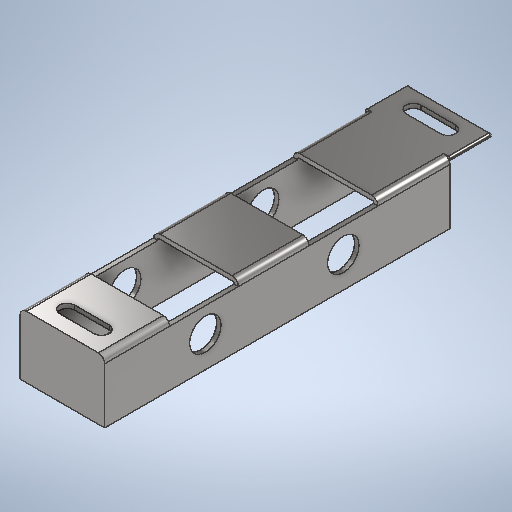
# Autodesk Inventor part: CASQUILLO RUEDA DE CORREDERA
Saved by Autodesk Inventor 2025 (Build 290162000, 162)
## iProperties
Created: 2026-02-25
Part Number: CASQUILLO RUEDA DE CORREDERA
Material: Acero inoxidable
Document SubType Name: Modeling
Designer: Frank
Density: 8 g/cm^3
Appearance: Semipulido
Author: Frank
Autodesk Inventor part; units mm, degrees
ref_plane "YZ Plane" through (0, 0, 0) normal (1, 0, 0) x (0, 1, 0)
ref_plane "XZ Plane" through (0, 0, 0) normal (0, 1, 0) x (-1, 0, 0)
ref_plane "XY Plane" through (0, 0, 0) normal (0, 0, 1) x (1, 0, 0)
sketch "Boceto1" plane through (0, 0, 0) normal (0, 0, 1) x (1, 0, 0)
  line L0 (0, 0) -> (0, 19.6)
  line L1 (0, 19.6) -> (-26.8, 19.6)
  line L2 (-26.8, 19.6) -> (-26.8, 0)
  line L3 (-25.4, 0) -> (-25.4, 18.2)
  line L4 (-25.4, 18.2) -> (-1.4, 18.2)
  line L5 (-1.4, 18.2) -> (-1.4, 0)
  line L6 (-26.8, 0) -> (-25.4, 0)
  line L7 (-1.4, 0) -> (0, 0)
  dimension "d1" = 19.6
  dimension "d2" = 1.4
  dimension "d4" = 26.8
  constraints: 16 end point, 4 perpendicular, 1 coincident, 1 collinear, 1 horizontal, 1 vertical, 2 other
  measures "d1" distance of L1.end L2.end
  measures "d2" distance between parallel lines of L4 L1
  measures "d4" distance of L0.end L1.end
extrude "Extrusión1" add sketch "Boceto1" against normal blind 108.4
fillet "Empalme1" radius 2 2 edges at (0, 19.6, -54.2) (-26.8, 19.6, -54.2)
ref_plane "Plano de trabajo1" through (0, 0, -108.4) normal (0, 0, -1) x (-1, 0, 0)
sketch "Boceto2" plane through (0, 0, -108.4) normal (0, 0, -1) x (-1, 0, 0)
  line L0 (0, 19.6) -> (26.8, 19.6)
  line L1 (26.8, 19.6) -> (26.8, 18.2)
  line L2 (26.8, 18.2) -> (0, 18.2)
  line L3 (0, 18.2) -> (0, 19.6)
  line L4 (26.8, 0) -> (26.8, 17.6) projected
  line L5 (0, 17.6) -> (0, 0) projected
  point P0 (1.4, 18.2)
  point P1 (2, 19.6)
  constraints: 8 end point, 2 collinear, 2 parallel, 2 point on line, 1 horizontal, 1 perpendicular
extrude "Extrusión2" add sketch "Boceto2" along normal blind 13.3
fillet "Empalme2" radius 0.5 1 edges at (-26.8, 18.2, -115.05)
fillet "Empalme3" radius 0.5 3 edges at (-26.8, 19.6, -115.05) (0, 19.6, -115.05) (0, 18.2, -115.05)
fillet "Empalme4" radius 0.5 8 edges at (-26.8, 18.9, -121.7) (-26.6536, 18.3464, -121.7) (-13.4, 18.2, -121.7) (-0.1464, 18.3464, -121.7) (0, 18.9, -121.7) (-0.1464, 19.4536, -121.7) (-13.4, 19.6, -121.7) (-26.6536, 19.4536, -121.7)
sketch "Boceto3" plane through (-24.8, 19.6, 0) normal (0, 1, 0) x (1, 0, 0)
  line L0 (5.91, 115.72) -> (16.89, 115.72) construction
  line L1 (5.91, 113.34) -> (16.89, 113.34)
  line L2 (16.89, 118.1) -> (5.91, 118.1)
  arc A0 (5.91, 118.1) -> (5.91, 113.34) centre (5.91, 115.72) ccw
  arc A1 (16.89, 113.34) -> (16.89, 118.1) centre (16.89, 115.72) ccw
  line L3 (-2, 121.2) -> (-2, 108.4) projected
  line L4 (24.3, 121.7) -> (-1.5, 121.7) projected
  line L5 (16.89, 5.98) -> (5.91, 5.98) construction
  line L6 (16.89, 3.6) -> (5.91, 3.6)
  line L7 (5.91, 8.36) -> (16.89, 8.36)
  arc A2 (16.89, 3.6) -> (16.89, 8.36) centre (16.89, 5.98) ccw
  arc A3 (5.91, 8.36) -> (5.91, 3.6) centre (5.91, 5.98) ccw
  line L8 (22.8, 0) -> (0, 0) projected
  line L9 (24.8, 0) -> (24.8, 108.4) projected
  point P0 (11.4, 115.72)
  point P1 (19.27, 115.72)
  point P2 (3.53, 115.72)
  point P3 (11.4, 5.98)
  point P4 (19.27, 5.98)
  point P5 (3.53, 5.98)
  dimension "d14" = 15.74
  dimension "d15" = 4.76
  dimension "d16" = 5.53
  dimension "d19" = 3.6
  dimension "d20" = 3.6
  dimension "d21" = 4.76
  dimension "d22" = 15.74
  dimension "d23" = 5.53
  constraints: 16 end point, 12 point on circle, 8 tangent, 4 centre point, 2 horizontal, 2 midpoint, 2 parallel
  measures "d14" distance of point (19.27, 115.72) point (3.53, 115.72)
  measures "d15" distance between parallel lines of L2 L1
  measures "d16" distance from line of L3 point (3.53, 115.72)
  measures "d19" distance between parallel lines of L4 L2
  measures "d20" distance between parallel lines of L8 L6
  measures "d21" distance between parallel lines of L6 L7
  measures "d22" distance of point (19.27, 5.98) point (3.53, 5.98)
  measures "d23" distance from line of L9 point (19.27, 5.98)
extrude "Extrusión3" cut sketch "Boceto3" against normal through all
ref_plane "Plano de trabajo2" through (0, 0, 0) normal (0, 0, 1) x (1, 0, 0)
sketch "Boceto4" plane through (0, 0, 0) normal (0, 0, 1) x (1, 0, 0)
  line L0 (0, 0) -> (0, 17.6) projected
  line L1 (-26.8, 19.6) -> (0, 19.6)
  line L2 (0, 19.6) -> (0, 0)
  line L3 (0, 0) -> (-26.8, 0)
  line L4 (-26.8, 0) -> (-26.8, 19.6)
  constraints: 8 end point, 2 parallel, 1 horizontal, 1 perpendicular
extrude "Extrusión4" add sketch "Boceto4" along normal blind 1
fillet "Empalme5" radius 2 2 edges at (0, 19.6, 0.5) (-26.8, 19.6, 0.5)
sketch "Boceto5" plane through (0, 0, -108.4) normal (1, 0, 0) x (0, 0, -1)
  circle A0 centre (-77.5, 9.8) radius 5
  circle A1 centre (-33.8, 9.8) radius 5
  line L0 (-109.4, 0) -> (-109.4, 17.6) projected
  line L1 (0, 0) -> (-109.4, 0) projected
  point P0 (-108.4, 0)
  dimension "d28" = 43.7
  dimension "d29" = 10
  dimension "d30" = 10
  dimension "d31" = 31.9
  dimension "d32" = 9.8
  dimension "d33" = 9.8
  constraints: 2 centre point
  measures "d28" distance of A1.centre A0.centre
  measures "d29" diameter of A0
  measures "d30" diameter of A1
  measures "d31" distance from line of L0 A0.centre
  measures "d32" distance from line of L1 A0.centre
  measures "d33" distance from line of L1 A1.centre
extrude "Extrusión5" cut sketch "Boceto5" against normal through all
ref_plane "Plano de trabajo3" through (-26.3, 19.6, -121.2) normal (0, 1, 0) x (1, 0, 0)
sketch "Boceto7" plane through (-26.3, 19.6, -121.2) normal (0, 1, 0) x (1, 0, 0)
  line L0 (26.3, -35.6145) -> (-0.5, -35.6145)
  line L1 (-0.5, -35.6145) -> (-0.5, -57.4145)
  line L2 (-0.5, -57.4145) -> (26.3, -57.4145)
  line L3 (26.3, -57.4145) -> (26.3, -35.6145)
  line L4 (26.3, -79.8455) -> (-0.5, -79.8455)
  line L5 (-0.5, -79.8455) -> (-0.5, -101.6455)
  line L6 (-0.5, -101.6455) -> (26.3, -101.6455)
  line L7 (26.3, -101.6455) -> (26.3, -79.8455)
  line L8 (26.3, -122.2) -> (26.3, -12.8) projected
  line L9 (-0.5, -12.8) -> (-0.5, -122.2) projected
  point P0 (26.3, -121.2)
  dimension "d37" = 21.8
  dimension "d38" = 21.8
  constraints: 16 end point, 4 parallel, 4 point on line, 2 horizontal, 2 perpendicular
  measures "d37" distance of L4.end L5.end
  measures "d38" distance of L0.end L1.end
extrude "Extrusión6" cut sketch "Boceto7" against normal blind 2 contours L3 L2 L1 L0 | L7 L6 L5 L4
